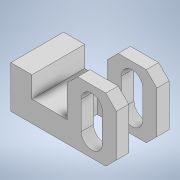
# Autodesk Inventor part: 14-2
Saved by Autodesk Inventor 2022 (Build 260153000, 153)
## iProperties
Created: 2021-09-12
Part Number: 14-2
Material: 일반
Document SubType Name: Modeling
Designer: 서울공업고등학교
Density: 1 g/cm^3
Appearance: 기본값
Author: 서울공업고등학교
Autodesk Inventor part; units mm, degrees
ref_plane "YZ Plane" through (0, 0, 0) normal (1, 0, 0) x (0, 1, 0)
ref_plane "XZ Plane" through (0, 0, 0) normal (0, 1, 0) x (-1, 0, 0)
ref_plane "XY Plane" through (0, 0, 0) normal (0, 0, 1) x (1, 0, 0)
sketch "스케치1" plane through (0, 0, 0) normal (0, 0, 1) x (1, 0, 0)
  line L0 (0, 0) -> (-14, 0)
  line L1 (-14, 6) -> (-14, 18)
  line L2 (-14, 18) -> (0, 18)
  line L3 (0, 18) -> (0, 0)
  line L4 (-14, 0) -> (-30, 0)
  line L5 (-30, 0) -> (-30, 12)
  line L6 (-30, 12) -> (-24, 12)
  line L7 (-24, 12) -> (-24, 6)
  line L8 (-24, 6) -> (-14, 6)
  line L9 (-7, 13) -> (-7, 5) construction
  line L10 (-10, 13) -> (-10, 5)
  line L11 (-4, 5) -> (-4, 13)
  arc A0 (-4, 13) -> (-10, 13) centre (-7, 13) ccw
  arc A1 (-10, 5) -> (-4, 5) centre (-7, 5) ccw
  point P0 (-7, 9)
  dimension "d0" = 14
  dimension "d3" = 12
  dimension "d4" = 6
  dimension "d5" = 10
  dimension "d6" = 30
  dimension "d7" = 6
  dimension "d8" = 8
  dimension "d9" = 5
  dimension "d10" = 7
  dimension "d11" = 18
  constraints: 26 end point, 5 perpendicular, 4 point on circle, 4 tangent, 3 parallel, 2 centre point, 2 horizontal, 1 midpoint, 1 vertical
  measures "d0" distance of L1.end L2.end
  measures "d3" distance of L4.end L5.end
  measures "d4" distance of L6.end L7.end
  measures "d5" distance of L1.start L7.end
  measures "d6" distance between parallel lines of L3 L5
  measures "d7" diameter of A1
  measures "d8" distance of L9.start L9.end
  measures "d9" distance from line of L0 L9.end
  measures "d10" distance from line of L3 L9.end
  measures "d11" distance between parallel lines of L0 L2
extrude "돌출1" add sketch "스케치1" along normal mid plane 15
chamfer "모따기1" distance 3 angle 45 3 edges at (-14, 18, 0) (0, 18, 0) (0, 0, 0)
sketch "스케치2" plane through (0, 0, 0) normal (0, 0, 1) x (1, 0, 0)
  line L0 (-17, 20.9368) -> (7.8455, 20.9368)
  line L1 (7.8455, 20.9368) -> (7.8455, -4.4634)
  line L2 (7.8455, -4.4634) -> (-17, -4.4634)
  line L3 (-17, -4.4634) -> (-17, 20.9368)
  line L4 (0, 15) -> (0, 3) projected
  point P0 (0, 0)
  dimension "d17" = 17
  constraints: 8 end point, 2 parallel, 1 horizontal, 1 perpendicular
  measures "d17" distance between parallel lines of L3 L4
extrude "돌출2" cut sketch "스케치2" along normal mid plane 8
